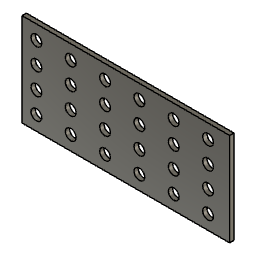
plate_2 v1 (Autodesk Fusion 360 design; units mm, degrees)
Autodesk Fusion 360 part; units mm, degrees
sketch "Sketch1" plane through (0, 0, 0) normal (0, 1, 0) x (1, 0, 0)
  line L0 (0, 0) -> (290.2, 0)
  line L1 (290.2, 0) -> (290.2, -130)
  line L2 (290.2, -130) -> (0, -130)
  line L3 (0, -130) -> (0, 0)
  dimension "d1" = 290.2
  dimension "d2" = 130
  constraint horizontal L0
  constraint vertical L1
  constraint horizontal L2
  constraint vertical L3
  constraint coincident L0.start L3.end
  measures "d1" distance of L0.start L0.end
  measures "d2" distance of L0.start L2.end
extrude "Extrude1" add sketch "Sketch1" against normal blind 6
sketch "Sketch2" plane through (0, -6, 0) normal (0, -1, 0) x (1, 0, 0)
  line L0 (290.2, 130) -> (0, 130)
  line L1 (0, 130) -> (0, 0)
  line L2 (0, 0) -> (290.2, 0)
  line L3 (290.2, 0) -> (290.2, 130)
  circle A0 centre (20, 110) radius 7.5
  circle A1 centre (68, 110) radius 7.5
  circle A2 centre (116, 110) radius 7.5
  circle A3 centre (164, 110) radius 7.5
  circle A4 centre (212, 110) radius 7.5
  circle A5 centre (260, 110) radius 7.5
  circle A6 centre (20, 80) radius 7.5
  circle A7 centre (68, 80) radius 7.5
  circle A8 centre (116, 80) radius 7.5
  circle A9 centre (164, 80) radius 7.5
  circle A10 centre (212, 80) radius 7.5
  circle A11 centre (260, 80) radius 7.5
  circle A12 centre (20, 50) radius 7.5
  circle A13 centre (68, 50) radius 7.5
  circle A14 centre (116, 50) radius 7.5
  circle A15 centre (164, 50) radius 7.5
  circle A16 centre (212, 50) radius 7.5
  circle A17 centre (260, 50) radius 7.5
  circle A18 centre (20, 20) radius 7.5
  circle A19 centre (68, 20) radius 7.5
  circle A20 centre (116, 20) radius 7.5
  circle A21 centre (164, 20) radius 7.5
  circle A22 centre (212, 20) radius 7.5
  circle A23 centre (260, 20) radius 7.5
  dimension "d5" = 15
  dimension "d6" = 20
  dimension "d7" = 20
  dimension "d10" = 240
  dimension "d11" = -90
  measures "d5" diameter of A0
  measures "d6" distance of L0 A0.centre
  measures "d7" distance of L1 A0.centre
extrude "Extrude2" cut sketch "Sketch2" against normal up to surface (6 mm away) contours A0 | A1 | A2 | A3 | A4 | A5 | A6 | A7 | A8 | A9 | A10 | A11 | A12 | A13 | A14 | A15 | A16 | A17 | A18 | A19 | A20 | A21 | A22 | A23
